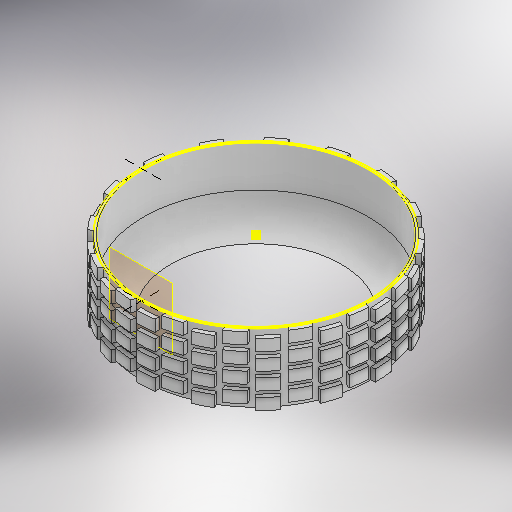
# Autodesk Inventor part: ridge_v2_treads
Saved by Autodesk Inventor 2026 (Build 300175050, 175E)
## iProperties
Created: 2026-06-28
Part Number: ridge_v2_treads
Material: Generic
Document SubType Name: Modeling
Designer: satom
Density: 1 g/cm^3
Appearance: Default
Author: satom
Autodesk Inventor part; units mm, degrees
note: some values were not read from the file. Chosen so that the rebuilt part matches the saved one: direction of "Emboss4".
ref_plane "YZ Plane" through (0, 0, 0) normal (1, 0, 0) x (0, 1, 0)
ref_plane "XZ Plane" through (0, 0, 0) normal (0, 1, 0) x (-1, 0, 0)
ref_plane "XY Plane" through (0, 0, 0) normal (0, 0, 1) x (1, 0, 0)
sketch "Sketch1" plane through (0, 0, 0) normal (0, 1, 0) x (-1, 0, 0)
  circle A0 centre (0, 0) radius 39.75
  circle A1 centre (0, 0) radius 40.5
  dimension "d0" = 79.5
  dimension "d1" = 81
  constraints: 2 centre point, 2 coincident
  measures "d0" diameter of A0
  measures "d1" diameter of A1
extrude "Extrusion1" add sketch "Sketch1" along normal blind 24
sketch "Sketch3" plane through (0, 24, 0) normal (0, 1, 0) x (1, 0, 0)
  circle A0 centre (0, 0) radius 40.5 projected
  circle A1 centre (0, 0) radius 39.75 projected
  point P0 (0, -40.5)
  point P1 (-39.75, 0)
  constraints: 1 horizontal alignment, 1 vertical alignment, 2 other
ref_plane "Work Plane2" through (0, 24, 40.5) normal (0, 0, 1) x (1, 0, 0)
sketch "Sketch7" plane through (0, 0, 0) normal (0, 0, 1) x (1, 0, 0)
  line L0 (39.75, 24) -> (39.75, 0) construction
  line L1 (0, 0) -> (-30, 0) construction
  line L2 (0, 0) -> (0, 12) construction
  line L3 (0, 12) -> (-39.75, 12) construction
  line L4 (0, 24) -> (-30, 24) construction
  ellipse E0 centre (0, 0.5748) end of major axis (-20.7169, 56.9851) minor radius 37.0729 (-40.5, 24) -> (-40.231, 12) ccw projected
  line L5 (-30, 0) -> (-40.5, 0)
  line L6 (-40.5, 24) -> (-40.5, 0)
  line L7 (-40.5, 12) -> (-37.9524, 12) construction
  line L8 (-40.5, 12) -> (-40.5, 13.6344) construction
  arc A0 (-39.6019, 9.6019) -> (-30, 0) centre (-30, 9.6019) ccw
  line L9 (-30, 0) -> (-30, 9.6019) construction
  line L10 (-39.6019, 9.6019) -> (-30, 9.6019) construction
  line L11 (-30, 24) -> (-30, 13.1677) construction
  line L12 (-40.8323, 13.1677) -> (-30, 13.1677) construction
  line L13 (0, -7.1864) -> (0, 29.1977) projected
  line L14 (-39.6019, 9.6019) -> (-39.6019, 0)
  point P0 (-39.5989, 9.3602)
  dimension "d24" = 30
  dimension "d25" = 12
  dimension "d26" = 39.75
  dimension "d27" = 30
  dimension "d28" = 90
  dimension "d29" = 90
  constraints: 26 end point, 3 horizontal, 3 point on line, 2 perpendicular, 2 point on circle, 2 vertical, 1 centre point, 1 midpoint, 1 tangent, 1 other
  measures "d24" distance of L1.start L1.end
  measures "d25" distance of L1.start L2.end
  measures "d26" distance of L2.end L3.end
  measures "d27" distance of L4.start L4.end
  measures "d28" angle of L10 L9
  measures "d29" angle of L11 L12
revolve "Revolution1" add sketch "Sketch7" angle 360 about axis through (0, -10, 0) along (0, 1, 0)
sketch "Sketch9" plane through (0, 24, 40.5) normal (0, 0, 1) x (1, 0, 0)
  line L0 (40.5, 0) -> (-40.5, 0) projected
  line L1 (0, -2) -> (6, -2)
  line L2 (6, -2) -> (6, -6)
  line L3 (6, -6) -> (0, -6)
  line L4 (0, -6) -> (0, -2)
  line L5 (8, 0) -> (14, 0)
  line L6 (14, 0) -> (14, -4)
  line L7 (14, -4) -> (8, -4)
  line L8 (8, -4) -> (8, 0)
  line L9 (40.5, -24) -> (-40.5, -24) projected
  line L10 (0, -8) -> (6, -8)
  line L11 (6, -8) -> (6, -12)
  line L12 (6, -12) -> (0, -12)
  line L13 (0, -12) -> (0, -8)
  line L14 (0, -14) -> (6, -14)
  line L15 (6, -14) -> (6, -18)
  line L16 (6, -18) -> (0, -18)
  line L17 (0, -18) -> (0, -14)
  line L18 (0, -20) -> (6, -20)
  line L19 (6, -20) -> (6, -24)
  line L20 (6, -24) -> (0, -24)
  line L21 (0, -24) -> (0, -20)
  line L22 (14, -10) -> (8, -10)
  line L23 (8, -6) -> (14, -6)
  line L24 (14, -6) -> (14, -10)
  line L25 (8, -10) -> (8, -6)
  line L26 (14, -16) -> (8, -16)
  line L27 (8, -12) -> (14, -12)
  line L28 (14, -12) -> (14, -16)
  line L29 (8, -16) -> (8, -12)
  line L30 (14, -22) -> (8, -22)
  line L31 (8, -18) -> (14, -18)
  line L32 (14, -18) -> (14, -22)
  line L33 (8, -22) -> (8, -18)
  point P0 (6, -7.8535)
  point P1 (8, -2)
  point P2 (6, -13.8535)
  point P3 (6, -19.8535)
  point P4 (6, -25.8535)
  point P5 (0, 0)
  point P6 (0, -4)
  point P7 (8, -8)
  point P8 (8, -14)
  point P9 (8, -20)
  dimension "d53" = 4
  dimension "d55" = 2
  dimension "d56" = 6
  dimension "d57" = 6
  dimension "d64" = 2
  dimension "d66" = 4
  dimension "d69" = 6
  dimension "d74" = 0
  dimension "d75" = 0
  dimension "d78" = 6
  constraints: 64 end point, 4 parallel, 4 point on line, 3 midpoint, 2 collinear, 2 horizontal, 2 perpendicular, 2 vertical, 52 other
  measures "d53" distance of L1.end L2.end
  measures "d55" distance from line of L2 point (8, -2)
  measures "d56" distance of L2.end L3.end
  measures "d57" distance of L5.start L5.end
  measures "d64" distance between parallel lines of L0 L1
  measures "d66" distance of L5.end L6.end
  measures "d69" distance of L2.end L11.end
  measures "d74" distance between parallel lines of L0 L5
  measures "d75" horizontal distance of point (0, 0) point (0, -4)
  measures "d78" distance of L6.end L22.start
emboss "Emboss4" sketch "Sketch9" operation add depth 1.5 direction (0, 0, -1)
pattern_circular "Circular Pattern5" count 16 over 360 about axis through (0, 0, 0) along (0, 1, 0) of "Emboss4"
equation "\"d57\" = d56"
body "Solid1"
